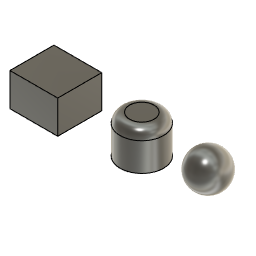
Custom appr (Autodesk Fusion 360 design; units mm, degrees)
Autodesk Fusion 360 part; units mm, degrees
sketch "Sketch1" plane through (0, 0, 0) normal (0, 0, 1) x (1, 0, 0)
  line L0 (-64.4967, -6.1848) -> (-13.9478, -6.1848)
  line L1 (-13.9478, -6.1848) -> (-13.9478, 40.4118)
  line L2 (-13.9478, 40.4118) -> (-64.4967, 40.4118)
  line L3 (-64.4967, 40.4118) -> (-64.4967, -6.1848)
  circle A0 centre (33.4809, 20.4418) radius 22.9427
  constraint horizontal L0
  constraint vertical L1
  constraint horizontal L2
  constraint vertical L3
extrude "Extrude1" add sketch "Sketch1" along normal blind 35 contours L0 L1 L2 L3 makes body 1
extrude "Extrude2" add sketch "Sketch1" along normal blind 40 separate body contours A0 makes body 2
sketch "Sketch2" plane through (0, 0, 0) normal (0, 0, 1) x (1, 0, 0)
  line L0 (105.8804, 23.2491) -> (105.8804, 43.2491)
  line L1 (105.8804, 23.2491) -> (105.8804, 3.2491)
  line L2 (105.8804, 43.2491) -> (105.8804, 53.1902) construction
  arc A0 (105.8804, 3.2491) -> (105.8804, 43.2491) centre (105.8804, 23.2491) ccw
  dimension "d5" = 40
  constraint coincident L0.start L1.start
  constraint vertical L0
  constraint parallel L0 L1
  constraint parallel L0 L2
  measures "d5" diameter of A0
revolve "Revolve1" add sketch "Sketch2" angle 360 about axis through (105.8804, 43.2491, 0) along (0, 1, 0) separate body makes body 3
move_body "MoveFace1" bodies 3 to x (1, 0, 0) y (0, 1, 0) z (0, 0, 1) at (10, 0, 20) on bodies 3
move_face "MoveFace2" to x (1, 0, 0) y (0, 1, 0) z (0, 0, 1) at (15, 0, 0) 1 faces at (56.3951, 19.2982, 26.6667) on bodies 2
fillet "Fillet1" radius 10 1 edges at (27.0908, 12.1454, 40) on bodies 2
